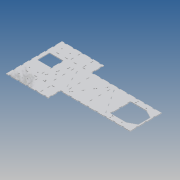
# Autodesk Inventor part: CaissonBase
Saved by Autodesk Inventor 2019 (Build 230136000, 136)
## iProperties
Created: 2019-08-26
Part Number: CaissonBase
Material: PVC-U
Document SubType Name: Modeling
Designer: jeremias.salamin
Density: 1.4 g/cm^3
Appearance: Lisse - Blanc
Description: CaissonBase
Mass: 70.9472 g
Surface Area: 655.131 cm^2
Volume: 50.6766 cm^3
Author: jeremias.salamin
Autodesk Inventor part; units mm, degrees
ref_plane "YZ Plane" through (0, 0, 0) normal (1, 0, 0) x (0, 1, 0)
ref_plane "XZ Plane" through (0, 0, 0) normal (0, 1, 0) x (-1, 0, 0)
ref_plane "XY Plane" through (0, 0, 0) normal (0, 0, 1) x (1, 0, 0)
sketch "Sketch1" plane through (0, 0, 0) normal (0, 0, 1) x (1, 0, 0)
  line L0 (0, 112) -> (0, -112) construction
  line L1 (-77.5006, 0) -> (370.4994, 0) construction
  line L2 (-13.5006, 0) -> (-13.5006, -80)
  line L3 (-13.5006, -80) -> (106.4994, -80)
  line L4 (106.4994, -80) -> (106.4994, -45)
  line L5 (106.4994, -45) -> (306.4994, -45)
  line L6 (306.4994, -45) -> (306.4994, 0)
  line L7 (-13.5006, 0) -> (-13.5006, 80)
  line L8 (-13.5006, 80) -> (106.4994, 80)
  line L9 (106.4994, 80) -> (106.4994, 45)
  line L10 (106.4994, 45) -> (306.4994, 45)
  line L11 (306.4994, 45) -> (306.4994, 0)
  point P0 (0, 0)
  dimension "d0" = 13.5006
  dimension "d1" = 80
  dimension "d2" = 120
  dimension "d3" = 200
  dimension "d4" = 45
  dimension "d5" = 320
  constraints: 20 end point, 4 symmetric about line, 2 perpendicular, 2 point on line, 1 parallel, 1 vertical
  measures "d0" distance between parallel lines of L7 L0
  measures "d1" distance of L2.start L2.end
  measures "d2" distance of L2.end L3.end
  measures "d3" distance of L4.end L5.end
  measures "d4" distance of L5.end L6.end
  measures "d5" distance between parallel lines of L2 L6
extrude "Extrusion1" add sketch "Sketch1" along normal mid plane 1.6
sketch "Esquisse2" plane through (0, 0, 0.8) normal (0, 0, 1) x (1, 0, 0)
  line L0 (-13.5006, 80) -> (-13.5006, -80) construction
  line L1 (-13.5006, -80) -> (106.4994, -80) construction
  line L2 (106.4994, -80) -> (106.4994, -45) construction
  line L3 (106.4994, -45) -> (306.4994, -45) construction
  line L4 (306.4994, -45) -> (306.4994, 45) construction
  line L5 (306.4994, 45) -> (106.4994, 45) construction
  line L6 (106.4994, 45) -> (106.4994, 80) construction
  line L7 (106.4994, 80) -> (-13.5006, 80) construction
  line L8 (0, 112) -> (0, -112) construction
  line L9 (-77.5006, 0) -> (370.4994, 0) construction
  arc A0 (278.9561, 15.2899) -> (278.9561, -15.2899) centre (255.4994, 0) ccw construction
  arc A1 (278.9561, -15.2899) -> (278.9561, 15.2899) centre (281.4994, 0) ccw construction
  line L10 (234.4994, 29.5) -> (279.4994, 29.5)
  line L11 (279.4994, -29.5) -> (234.4994, -29.5)
  line L12 (234.4994, -29.5) -> (234.4994, 29.5)
  line L13 (302.4994, -17.5) -> (302.4994, 17.5)
  line L14 (279.4994, 29.5) -> (302.4994, 17.5)
  line L15 (302.4994, -17.5) -> (279.4994, -29.5)
  point P0 (0, 0)
  dimension "d8" = 56
  dimension "d9" = 31
  dimension "d10" = 26
  dimension "d11" = 25
  dimension "d12" = 59
  dimension "d13" = 35
  dimension "d15" = 45
  dimension "d16" = 4
  dimension "d23" = 117.553
  dimension "d24" = 117.553
  dimension "d25" = 25.9422
  dimension "d62" = 27
  constraints: 12 end point, 4 point on circle, 2 centre point, 2 point on line, 1 horizontal, 1 parallel, 1 other
  measures "d8" diameter of A0
  measures "d9" diameter of A1
  measures "d10" distance of A1.centre A0.centre
  measures "d11" distance from line of L4 A1.centre
  measures "d12" distance of L11.end L10.start
  measures "d13" distance of L13.start L13.end
  measures "d15" distance of L10.start L10.end
  measures "d16" distance between parallel lines of L4 L13
  measures "d23" angle of L13 L14
  measures "d24" angle of L13 L15
  measures "d25" distance of L13.start L11.start
  measures "d62" distance from line of L4 L10.end
extrude "Extrusion2" cut sketch "Esquisse2" against normal through all
sketch "Esquisse3" plane through (0, 0, 0.8) normal (0, 0, 1) x (1, 0, 0)
  line L0 (234.4994, -29.5) -> (234.4994, 29.5) construction
  line L1 (234.4994, 29.5) -> (279.4994, 29.5) construction
  line L2 (279.4994, 29.5) -> (302.4994, 17.5) construction
  line L3 (302.4994, 17.5) -> (302.4994, -17.5) construction
  line L4 (302.4994, -17.5) -> (279.4994, -29.5) construction
  line L5 (279.4994, -29.5) -> (234.4994, -29.5) construction
  line L6 (-13.5006, 80) -> (-13.5006, -80) construction
  line L7 (-13.5006, -80) -> (106.4994, -80) construction
  line L8 (106.4994, -80) -> (106.4994, -45) construction
  line L9 (106.4994, -45) -> (306.4994, -45) construction
  line L10 (306.4994, -45) -> (306.4994, 45) construction
  line L11 (306.4994, 45) -> (106.4994, 45) construction
  line L12 (106.4994, 45) -> (106.4994, 80) construction
  line L13 (106.4994, 80) -> (-13.5006, 80) construction
  line L14 (0, 112) -> (0, -112) construction
  line L15 (-77.5006, 0) -> (370.4994, 0) construction
  point P0 (0, 0)
  point P1 (272.9994, 35)
  point P2 (272.9994, -35)
  dimension "d26" = 33.5
  dimension "d45" = 70
  constraints: 1 symmetric about line
  measures "d26" distance from line of point (272.999, 35) L10
  measures "d45" distance of point (272.999, -35) point (272.999, 35)
hole "Perçage3" at (272.9994, 35, 0.8) at (272.9994, -35, 0.8) direction (0, 0, -1) diameter 3 end through all
sketch "Esquisse4" plane through (0, 0, 0.8) normal (0, 0, 1) x (1, 0, 0)
  circle A0 centre (272.9994, 35) radius 1.5 construction
  circle A1 centre (272.9994, -35) radius 1.5 construction
  line L0 (234.4994, -29.5) -> (234.4994, 29.5) construction
  line L1 (234.4994, 29.5) -> (279.4994, 29.5) construction
  line L2 (279.4994, 29.5) -> (302.4994, 17.5) construction
  line L3 (302.4994, 17.5) -> (302.4994, -17.5) construction
  line L4 (302.4994, -17.5) -> (279.4994, -29.5) construction
  line L5 (279.4994, -29.5) -> (234.4994, -29.5) construction
  line L6 (-13.5006, 80) -> (-13.5006, -80) construction
  line L7 (-13.5006, -80) -> (106.4994, -80) construction
  line L8 (106.4994, -80) -> (106.4994, -45) construction
  line L9 (106.4994, -45) -> (306.4994, -45) construction
  line L10 (306.4994, -45) -> (306.4994, 45) construction
  line L11 (306.4994, 45) -> (106.4994, 45) construction
  line L12 (106.4994, 45) -> (106.4994, 80) construction
  line L13 (106.4994, 80) -> (-13.5006, 80) construction
  line L14 (0, 112) -> (0, -112) construction
  line L15 (-77.5006, 0) -> (370.4994, 0) construction
  line L16 (-3.5006, 34) -> (36.4994, 34)
  line L17 (36.4994, 34) -> (36.4994, -1.4)
  line L18 (36.4994, -1.4) -> (-3.5006, -1.4)
  line L19 (-3.5006, -1.4) -> (-3.5006, 34)
  point P0 (0, 0)
  dimension "d56" = 35.4
  dimension "d57" = 78.6
  dimension "d58" = 10
  dimension "d59" = 40
  constraints: 8 end point, 2 parallel, 1 horizontal, 1 perpendicular
  measures "d56" distance between parallel lines of L16 L18
  measures "d57" distance between parallel lines of L7 L18
  measures "d58" distance between parallel lines of L6 L19
  measures "d59" distance between parallel lines of L17 L19
extrude "Extrusion3" cut sketch "Esquisse4" against normal through all
sketch "Esquisse5" plane through (0, 0, 0.8) normal (0, 0, 1) x (1, 0, 0)
  line L0 (-3.5006, -1.4) -> (-3.5006, 34) construction
  line L1 (-3.5006, 34) -> (36.4994, 34) construction
  line L2 (36.4994, 34) -> (36.4994, -1.4) construction
  line L3 (36.4994, -1.4) -> (-3.5006, -1.4) construction
  circle A0 centre (272.9994, 35) radius 1.5 construction
  circle A1 centre (272.9994, -35) radius 1.5 construction
  line L4 (234.4994, -29.5) -> (234.4994, 29.5) construction
  line L5 (234.4994, 29.5) -> (279.4994, 29.5) construction
  line L6 (279.4994, 29.5) -> (302.4994, 17.5) construction
  line L7 (302.4994, 17.5) -> (302.4994, -17.5) construction
  line L8 (302.4994, -17.5) -> (279.4994, -29.5) construction
  line L9 (279.4994, -29.5) -> (234.4994, -29.5) construction
  line L10 (-13.5006, 80) -> (-13.5006, -80) construction
  line L11 (-13.5006, -80) -> (106.4994, -80) construction
  line L12 (106.4994, -80) -> (106.4994, -45) construction
  line L13 (106.4994, -45) -> (306.4994, -45) construction
  line L14 (306.4994, -45) -> (306.4994, 45) construction
  line L15 (306.4994, 45) -> (106.4994, 45) construction
  line L16 (106.4994, 45) -> (106.4994, 80) construction
  line L17 (106.4994, 80) -> (-13.5006, 80) construction
  line L18 (0, 112) -> (0, -112) construction
  line L19 (-77.5006, 0) -> (370.4994, 0) construction
  point P0 (0, 0)
  point P1 (4.4994, 61.4)
  point P2 (28.4994, 61.4)
  point P3 (4.4994, -61.4)
  point P4 (28.4994, -61.4)
  point P5 (4.4994, -31.4)
  point P6 (28.4994, -31.4)
  dimension "d63" = 18.6
  dimension "d64" = 18.6
  dimension "d65" = 24
  dimension "d66" = 18
  dimension "d67" = 30
  dimension "d68" = 30
  dimension "d69" = 24
  dimension "d70" = 18
  constraints: 2 symmetric about line
  measures "d63" distance from line of L17 point (4.499, 61.4)
  measures "d64" distance from line of L17 point (28.499, 61.4)
  measures "d65" distance of point (28.499, 61.4) point (4.499, 61.4)
  measures "d66" distance from line of point (4.499, 61.4) L10
  measures "d67" distance of point (4.499, -61.4) point (4.499, -31.4)
  measures "d68" distance of point (28.499, -61.4) point (28.499, -31.4)
  measures "d69" distance of point (4.499, -31.4) point (28.499, -31.4)
  measures "d70" distance from line of L10 point (4.499, -31.4)
hole "Perçage4" at (4.4994, 61.4, 0.8) at (28.4994, 61.4, 0.8) at (4.4994, -61.4, 0.8) at (28.4994, -61.4, 0.8) at (4.4994, -31.4, 0.8) at (28.4994, -31.4, 0.8) direction (0, 0, -1) diameter 3 end through all
sketch "Esquisse6" plane through (0, 0, 0.8) normal (0, 0, 1) x (1, 0, 0)
  circle A0 centre (4.4994, -31.4) radius 1.5 construction
  circle A1 centre (4.4994, -61.4) radius 1.5 construction
  circle A2 centre (4.4994, 61.4) radius 1.5 construction
  circle A3 centre (28.4994, 61.4) radius 1.5 construction
  circle A4 centre (28.4994, -61.4) radius 1.5 construction
  circle A5 centre (28.4994, -31.4) radius 1.5 construction
  line L0 (-3.5006, -1.4) -> (-3.5006, 34) construction
  line L1 (-3.5006, 34) -> (36.4994, 34) construction
  line L2 (36.4994, 34) -> (36.4994, -1.4) construction
  line L3 (36.4994, -1.4) -> (-3.5006, -1.4) construction
  circle A6 centre (272.9994, 35) radius 1.5 construction
  circle A7 centre (272.9994, -35) radius 1.5 construction
  line L4 (234.4994, -29.5) -> (234.4994, 29.5) construction
  line L5 (234.4994, 29.5) -> (279.4994, 29.5) construction
  line L6 (279.4994, 29.5) -> (302.4994, 17.5) construction
  line L7 (302.4994, 17.5) -> (302.4994, -17.5) construction
  line L8 (302.4994, -17.5) -> (279.4994, -29.5) construction
  line L9 (279.4994, -29.5) -> (234.4994, -29.5) construction
  line L10 (-13.5006, 80) -> (-13.5006, -80) construction
  line L11 (-13.5006, -80) -> (106.4994, -80) construction
  line L12 (106.4994, -80) -> (106.4994, -45) construction
  line L13 (106.4994, -45) -> (306.4994, -45) construction
  line L14 (306.4994, -45) -> (306.4994, 45) construction
  line L15 (306.4994, 45) -> (106.4994, 45) construction
  line L16 (106.4994, 45) -> (106.4994, 80) construction
  line L17 (106.4994, 80) -> (-13.5006, 80) construction
  line L18 (0, 112) -> (0, -112) construction
  line L19 (-77.5006, 0) -> (370.4994, 0) construction
  point P0 (0, 0)
  point P1 (244.4994, 40)
  point P2 (244.4994, -40)
  dimension "d78" = 5
  dimension "d79" = 62
  constraints: 1 symmetric about line
  measures "d78" distance from line of L15 point (244.499, 40)
  measures "d79" distance from line of L14 point (244.499, 40)
hole "Perçage5" at (244.4994, 40, 0.8) at (244.4994, -40, 0.8) direction (0, 0, -1) diameter 3 end through all
sketch "Esquisse7" plane through (0, 0, 0.8) normal (0, 0, 1) x (1, 0, 0)
  circle A0 centre (244.4994, 40) radius 1.5 construction
  circle A1 centre (244.4994, -40) radius 1.5 construction
  circle A2 centre (4.4994, -31.4) radius 1.5 construction
  circle A3 centre (4.4994, -61.4) radius 1.5 construction
  circle A4 centre (4.4994, 61.4) radius 1.5 construction
  circle A5 centre (28.4994, 61.4) radius 1.5 construction
  circle A6 centre (28.4994, -61.4) radius 1.5 construction
  circle A7 centre (28.4994, -31.4) radius 1.5 construction
  line L0 (-3.5006, -1.4) -> (-3.5006, 34) construction
  line L1 (-3.5006, 34) -> (36.4994, 34) construction
  line L2 (36.4994, 34) -> (36.4994, -1.4) construction
  line L3 (36.4994, -1.4) -> (-3.5006, -1.4) construction
  circle A8 centre (272.9994, 35) radius 1.5 construction
  circle A9 centre (272.9994, -35) radius 1.5 construction
  line L4 (234.4994, -29.5) -> (234.4994, 29.5) construction
  line L5 (234.4994, 29.5) -> (279.4994, 29.5) construction
  line L6 (279.4994, 29.5) -> (302.4994, 17.5) construction
  line L7 (302.4994, 17.5) -> (302.4994, -17.5) construction
  line L8 (302.4994, -17.5) -> (279.4994, -29.5) construction
  line L9 (279.4994, -29.5) -> (234.4994, -29.5) construction
  line L10 (-13.5006, 80) -> (-13.5006, -80) construction
  line L11 (-13.5006, -80) -> (106.4994, -80) construction
  line L12 (106.4994, -80) -> (106.4994, -45) construction
  line L13 (106.4994, -45) -> (306.4994, -45) construction
  line L14 (306.4994, -45) -> (306.4994, 45) construction
  line L15 (306.4994, 45) -> (106.4994, 45) construction
  line L16 (106.4994, 45) -> (106.4994, 80) construction
  line L17 (106.4994, 80) -> (-13.5006, 80) construction
  line L18 (-77.5006, 0) -> (370.4994, 0) construction
  line L19 (0, 112) -> (0, -112) construction
  point P0 (0, 0)
  point P1 (244.4994, 33.4)
  point P2 (244.4994, -33.4)
  dimension "d87" = 11.6
  dimension "d88" = 62
  constraints: 1 symmetric about line
  measures "d87" distance from line of L15 point (244.499, 33.4)
  measures "d88" distance from line of L14 point (244.499, 33.4)
hole "Perçage6" at (244.4994, 33.4, 0.8) at (244.4994, -33.4, 0.8) direction (0, 0, -1) diameter 4 end through all
sketch "Esquisse10" plane through (0, 0, -0.8) normal (0, 0, -1) x (-1, 0, 0)
  line L0 (-75.4994, -80) -> (-75.4994, -78.4)
  line L1 (-75.4994, -78.4) -> (-67.4994, -78.4)
  line L2 (-67.4994, -78.4) -> (-67.4994, -80)
  line L3 (-67.4994, -80) -> (-75.4994, -80)
  line L4 (-25.4994, -80) -> (-25.4994, -78.4)
  line L5 (-25.4994, -78.4) -> (-17.4994, -78.4)
  line L6 (-17.4994, -78.4) -> (-17.4994, -80)
  line L7 (-17.4994, -80) -> (-25.4994, -80)
  line L8 (7.5006, -78.4) -> (7.5006, -80)
  line L9 (7.5006, -80) -> (-0.4994, -80)
  line L10 (-0.4994, -80) -> (-0.4994, -78.4)
  line L11 (-0.4994, -78.4) -> (7.5006, -78.4)
  line L12 (-50.4994, -80) -> (-50.4994, -78.4)
  line L13 (-50.4994, -78.4) -> (-42.4994, -78.4)
  line L14 (-42.4994, -78.4) -> (-42.4994, -80)
  line L15 (-42.4994, -80) -> (-50.4994, -80)
  line L16 (-100.4994, -80) -> (-100.4994, -78.4)
  line L17 (-100.4994, -78.4) -> (-92.4994, -78.4)
  line L18 (-92.4994, -78.4) -> (-92.4994, -80)
  line L19 (-92.4994, -80) -> (-100.4994, -80)
  line L20 (-255.7994, -43.4) -> (-255.7994, -45)
  line L21 (-255.7994, -45) -> (-263.7994, -45)
  line L22 (-263.7994, -45) -> (-263.7994, -43.4)
  line L23 (-263.7994, -43.4) -> (-255.7994, -43.4)
  line L24 (-205.7994, -43.4) -> (-205.7994, -45)
  line L25 (-205.7994, -45) -> (-213.7994, -45)
  line L26 (-213.7994, -45) -> (-213.7994, -43.4)
  line L27 (-213.7994, -43.4) -> (-205.7994, -43.4)
  line L28 (-155.7994, -43.4) -> (-155.7994, -45)
  line L29 (-155.7994, -45) -> (-163.7994, -45)
  line L30 (-163.7994, -45) -> (-163.7994, -43.4)
  line L31 (-163.7994, -43.4) -> (-155.7994, -43.4)
  line L32 (-105.7994, -43.4) -> (-105.7994, -45)
  line L33 (-105.7994, -45) -> (-113.7994, -45)
  line L34 (-113.7994, -45) -> (-113.7994, -43.4)
  line L35 (-113.7994, -43.4) -> (-105.7994, -43.4)
  line L36 (-55.7994, -43.4) -> (-55.7994, -45)
  line L37 (-55.7994, -45) -> (-63.7994, -45)
  line L38 (-63.7994, -45) -> (-63.7994, -43.4)
  line L39 (-63.7994, -43.4) -> (-55.7994, -43.4)
  line L40 (-5.7994, -43.4) -> (-5.7994, -45)
  line L41 (-5.7994, -45) -> (-13.7994, -45)
  line L42 (-13.7994, -45) -> (-13.7994, -43.4)
  line L43 (-13.7994, -43.4) -> (-5.7994, -43.4)
  line L44 (-30.7994, -43.4) -> (-30.7994, -45)
  line L45 (-30.7994, -45) -> (-38.7994, -45)
  line L46 (-38.7994, -45) -> (-38.7994, -43.4)
  line L47 (-38.7994, -43.4) -> (-30.7994, -43.4)
  line L48 (-80.7994, -43.4) -> (-80.7994, -45)
  line L49 (-80.7994, -45) -> (-88.7994, -45)
  line L50 (-88.7994, -45) -> (-88.7994, -43.4)
  line L51 (-88.7994, -43.4) -> (-80.7994, -43.4)
  line L52 (-130.7994, -43.4) -> (-130.7994, -45)
  line L53 (-130.7994, -45) -> (-138.7994, -45)
  line L54 (-138.7994, -45) -> (-138.7994, -43.4)
  line L55 (-138.7994, -43.4) -> (-130.7994, -43.4)
  line L56 (-180.7994, -43.4) -> (-180.7994, -45)
  line L57 (-180.7994, -45) -> (-188.7994, -45)
  line L58 (-188.7994, -45) -> (-188.7994, -43.4)
  line L59 (-188.7994, -43.4) -> (-180.7994, -43.4)
  line L60 (-230.7994, -43.4) -> (-230.7994, -45)
  line L61 (-230.7994, -45) -> (-238.7994, -45)
  line L62 (-238.7994, -45) -> (-238.7994, -43.4)
  line L63 (-238.7994, -43.4) -> (-230.7994, -43.4)
  line L64 (-280.7994, -43.4) -> (-280.7994, -45)
  line L65 (-280.7994, -45) -> (-288.7994, -45)
  line L66 (-288.7994, -45) -> (-288.7994, -43.4)
  line L67 (-288.7994, -43.4) -> (-280.7994, -43.4)
  line L68 (13.5006, 30.5) -> (11.9006, 30.5)
  line L69 (11.9006, 30.5) -> (11.9006, 38.5)
  line L70 (11.9006, 38.5) -> (13.5006, 38.5)
  line L71 (13.5006, 38.5) -> (13.5006, 30.5)
  line L72 (13.5006, -15.5) -> (11.9006, -15.5)
  line L73 (11.9006, -15.5) -> (11.9006, -7.5)
  line L74 (11.9006, -7.5) -> (13.5006, -7.5)
  line L75 (13.5006, -7.5) -> (13.5006, -15.5)
  line L76 (13.5006, -61.5) -> (11.9006, -61.5)
  line L77 (11.9006, -61.5) -> (11.9006, -53.5)
  line L78 (11.9006, -53.5) -> (13.5006, -53.5)
  line L79 (13.5006, -53.5) -> (13.5006, -61.5)
  line L80 (13.5006, -38.5) -> (11.9006, -38.5)
  line L81 (11.9006, -38.5) -> (11.9006, -30.5)
  line L82 (11.9006, -30.5) -> (13.5006, -30.5)
  line L83 (13.5006, -30.5) -> (13.5006, -38.5)
  line L84 (13.5006, 7.5) -> (11.9006, 7.5)
  line L85 (11.9006, 7.5) -> (11.9006, 15.5)
  line L86 (11.9006, 15.5) -> (13.5006, 15.5)
  line L87 (13.5006, 15.5) -> (13.5006, 7.5)
  line L88 (13.5006, 53.5) -> (11.9006, 53.5)
  line L89 (11.9006, 53.5) -> (11.9006, 61.5)
  line L90 (11.9006, 61.5) -> (13.5006, 61.5)
  line L91 (13.5006, 61.5) -> (13.5006, 53.5)
  line L92 (-104.8994, -75.7) -> (-106.4994, -75.7)
  line L93 (-106.4994, -75.7) -> (-106.4994, -67.7)
  line L94 (-106.4994, -67.7) -> (-104.8994, -67.7)
  line L95 (-104.8994, -67.7) -> (-104.8994, -75.7)
  line L96 (-104.8994, -55.7) -> (-106.4994, -55.7)
  line L97 (-106.4994, -55.7) -> (-106.4994, -47.7)
  line L98 (-106.4994, -47.7) -> (-104.8994, -47.7)
  line L99 (-104.8994, -47.7) -> (-104.8994, -55.7)
  line L100 (-304.8994, -4) -> (-306.4994, -4)
  line L101 (-306.4994, -4) -> (-306.4994, 4)
  line L102 (-306.4994, 4) -> (-304.8994, 4)
  line L103 (-304.8994, 4) -> (-304.8994, -4)
  line L104 (-304.8994, -29) -> (-306.4994, -29)
  line L105 (-306.4994, -29) -> (-306.4994, -21)
  line L106 (-306.4994, -21) -> (-304.8994, -21)
  line L107 (-304.8994, -21) -> (-304.8994, -29)
  line L108 (-304.8994, 21) -> (-306.4994, 21)
  line L109 (-306.4994, 21) -> (-306.4994, 29)
  line L110 (-306.4994, 29) -> (-304.8994, 29)
  line L111 (-304.8994, 29) -> (-304.8994, 21)
  line L112 (-255.7994, 45) -> (-255.7994, 43.4)
  line L113 (-255.7994, 43.4) -> (-263.7994, 43.4)
  line L114 (-263.7994, 43.4) -> (-263.7994, 45)
  line L115 (-263.7994, 45) -> (-255.7994, 45)
  line L116 (-205.7994, 45) -> (-205.7994, 43.4)
  line L117 (-205.7994, 43.4) -> (-213.7994, 43.4)
  line L118 (-213.7994, 43.4) -> (-213.7994, 45)
  line L119 (-213.7994, 45) -> (-205.7994, 45)
  line L120 (-155.7994, 45) -> (-155.7994, 43.4)
  line L121 (-155.7994, 43.4) -> (-163.7994, 43.4)
  line L122 (-163.7994, 43.4) -> (-163.7994, 45)
  line L123 (-163.7994, 45) -> (-155.7994, 45)
  line L124 (-105.7994, 45) -> (-105.7994, 43.4)
  line L125 (-105.7994, 43.4) -> (-113.7994, 43.4)
  line L126 (-113.7994, 43.4) -> (-113.7994, 45)
  line L127 (-113.7994, 45) -> (-105.7994, 45)
  line L128 (-55.7994, 45) -> (-55.7994, 43.4)
  line L129 (-55.7994, 43.4) -> (-63.7994, 43.4)
  line L130 (-63.7994, 43.4) -> (-63.7994, 45)
  line L131 (-63.7994, 45) -> (-55.7994, 45)
  line L132 (-5.7994, 45) -> (-5.7994, 43.4)
  line L133 (-5.7994, 43.4) -> (-13.7994, 43.4)
  line L134 (-13.7994, 43.4) -> (-13.7994, 45)
  line L135 (-13.7994, 45) -> (-5.7994, 45)
  line L136 (-30.7994, 45) -> (-30.7994, 43.4)
  line L137 (-30.7994, 43.4) -> (-38.7994, 43.4)
  line L138 (-38.7994, 43.4) -> (-38.7994, 45)
  line L139 (-38.7994, 45) -> (-30.7994, 45)
  line L140 (-80.7994, 45) -> (-80.7994, 43.4)
  line L141 (-80.7994, 43.4) -> (-88.7994, 43.4)
  line L142 (-88.7994, 43.4) -> (-88.7994, 45)
  line L143 (-88.7994, 45) -> (-80.7994, 45)
  line L144 (-130.7994, 45) -> (-130.7994, 43.4)
  line L145 (-130.7994, 43.4) -> (-138.7994, 43.4)
  line L146 (-138.7994, 43.4) -> (-138.7994, 45)
  line L147 (-138.7994, 45) -> (-130.7994, 45)
  line L148 (-180.7994, 45) -> (-180.7994, 43.4)
  line L149 (-180.7994, 43.4) -> (-188.7994, 43.4)
  line L150 (-188.7994, 43.4) -> (-188.7994, 45)
  line L151 (-188.7994, 45) -> (-180.7994, 45)
  line L152 (-230.7994, 45) -> (-230.7994, 43.4)
  line L153 (-230.7994, 43.4) -> (-238.7994, 43.4)
  line L154 (-238.7994, 43.4) -> (-238.7994, 45)
  line L155 (-238.7994, 45) -> (-230.7994, 45)
  line L156 (-280.7994, 45) -> (-280.7994, 43.4)
  line L157 (-280.7994, 43.4) -> (-288.7994, 43.4)
  line L158 (-288.7994, 43.4) -> (-288.7994, 45)
  line L159 (-288.7994, 45) -> (-280.7994, 45)
  line L160 (-104.8994, 47.7) -> (-106.4994, 47.7)
  line L161 (-106.4994, 47.7) -> (-106.4994, 55.7)
  line L162 (-106.4994, 55.7) -> (-104.8994, 55.7)
  line L163 (-104.8994, 55.7) -> (-104.8994, 47.7)
  line L164 (-104.8994, 67.7) -> (-106.4994, 67.7)
  line L165 (-106.4994, 67.7) -> (-106.4994, 75.7)
  line L166 (-106.4994, 75.7) -> (-104.8994, 75.7)
  line L167 (-104.8994, 75.7) -> (-104.8994, 67.7)
  line L168 (-75.4994, 78.4) -> (-75.4994, 80)
  line L169 (-75.4994, 80) -> (-67.4994, 80)
  line L170 (-67.4994, 80) -> (-67.4994, 78.4)
  line L171 (-67.4994, 78.4) -> (-75.4994, 78.4)
  line L172 (-25.4994, 78.4) -> (-25.4994, 80)
  line L173 (-25.4994, 80) -> (-17.4994, 80)
  line L174 (-17.4994, 80) -> (-17.4994, 78.4)
  line L175 (-17.4994, 78.4) -> (-25.4994, 78.4)
  line L176 (7.5006, 80) -> (7.5006, 78.4)
  line L177 (7.5006, 78.4) -> (-0.4994, 78.4)
  line L178 (-0.4994, 78.4) -> (-0.4994, 80)
  line L179 (-0.4994, 80) -> (7.5006, 80)
  line L180 (-50.4994, 78.4) -> (-50.4994, 80)
  line L181 (-50.4994, 80) -> (-42.4994, 80)
  line L182 (-42.4994, 80) -> (-42.4994, 78.4)
  line L183 (-42.4994, 78.4) -> (-50.4994, 78.4)
  line L184 (-100.4994, 78.4) -> (-100.4994, 80)
  line L185 (-100.4994, 80) -> (-92.4994, 80)
  line L186 (-92.4994, 80) -> (-92.4994, 78.4)
  line L187 (-92.4994, 78.4) -> (-100.4994, 78.4)
  line L188 (-44.6994, 75.7) -> (-43.0994, 75.7)
  line L189 (-43.0994, 75.7) -> (-43.0994, 67.7)
  line L190 (-43.0994, 67.7) -> (-44.6994, 67.7)
  line L191 (-44.6994, 67.7) -> (-44.6994, 75.7)
  line L192 (-44.6994, 55.7) -> (-43.0994, 55.7)
  line L193 (-43.0994, 55.7) -> (-43.0994, 47.7)
  line L194 (-43.0994, 47.7) -> (-44.6994, 47.7)
  line L195 (-44.6994, 47.7) -> (-44.6994, 55.7)
  line L196 (-81.2994, 75.7) -> (-79.6994, 75.7)
  line L197 (-79.6994, 75.7) -> (-79.6994, 67.7)
  line L198 (-79.6994, 67.7) -> (-81.2994, 67.7)
  line L199 (-81.2994, 67.7) -> (-81.2994, 75.7)
  line L200 (-81.2994, 55.7) -> (-79.6994, 55.7)
  line L201 (-79.6994, 55.7) -> (-79.6994, 47.7)
  line L202 (-79.6994, 47.7) -> (-81.2994, 47.7)
  line L203 (-81.2994, 47.7) -> (-81.2994, 55.7)
  line L204 (-93.3693, 4.9446) -> (-91.9076, 4.2939)
  line L205 (-91.9076, 4.2939) -> (-95.1615, -3.0145)
  line L206 (-95.1615, -3.0145) -> (-96.6232, -2.3637)
  line L207 (-96.6232, -2.3637) -> (-93.3693, 4.9446)
  line L208 (-83.2009, 27.7833) -> (-81.7392, 27.1325)
  line L209 (-81.7392, 27.1325) -> (-84.9931, 19.8241)
  line L210 (-84.9931, 19.8241) -> (-86.4548, 20.4749)
  line L211 (-86.4548, 20.4749) -> (-83.2009, 27.7833)
  line L212 (-103.5377, -17.894) -> (-102.0761, -18.5448)
  line L213 (-102.0761, -18.5448) -> (-105.3299, -25.8531)
  line L214 (-105.3299, -25.8531) -> (-106.7916, -25.2024)
  line L215 (-106.7916, -25.2024) -> (-103.5377, -17.894)
  line L216 (-72.2994, 4) -> (-70.6994, 4)
  line L217 (-70.6994, 4) -> (-70.6994, -4)
  line L218 (-70.6994, -4) -> (-72.2994, -4)
  line L219 (-72.2994, -4) -> (-72.2994, 4)
  line L220 (-72.2994, 29) -> (-70.6994, 29)
  line L221 (-70.6994, 29) -> (-70.6994, 21)
  line L222 (-70.6994, 21) -> (-72.2994, 21)
  line L223 (-72.2994, 21) -> (-72.2994, 29)
  line L224 (-72.2994, -21) -> (-70.6994, -21)
  line L225 (-70.6994, -21) -> (-70.6994, -29)
  line L226 (-70.6994, -29) -> (-72.2994, -29)
  line L227 (-72.2994, -29) -> (-72.2994, -21)
  line L228 (-52.4477, -3.9304) -> (-53.9605, -4.4513)
  line L229 (-53.9605, -4.4513) -> (-56.5651, 3.1128)
  line L230 (-56.5651, 3.1128) -> (-55.0522, 3.6337)
  line L231 (-55.0522, 3.6337) -> (-52.4477, -3.9304)
  line L232 (-44.3085, -27.5684) -> (-45.8213, -28.0893)
  line L233 (-45.8213, -28.0893) -> (-48.4259, -20.5251)
  line L234 (-48.4259, -20.5251) -> (-46.913, -20.0042)
  line L235 (-46.913, -20.0042) -> (-44.3085, -27.5684)
  line L236 (-60.5869, 19.7076) -> (-62.0997, 19.1866)
  line L237 (-62.0997, 19.1866) -> (-64.7043, 26.7508)
  line L238 (-64.7043, 26.7508) -> (-63.1914, 27.2717)
  line L239 (-63.1914, 27.2717) -> (-60.5869, 19.7076)
  line L240 (-38.0994, 4) -> (-36.4994, 4)
  line L241 (-36.4994, 4) -> (-36.4994, -4)
  line L242 (-36.4994, -4) -> (-38.0994, -4)
  line L243 (-38.0994, -4) -> (-38.0994, 4)
  line L244 (-38.0994, 29) -> (-36.4994, 29)
  line L245 (-36.4994, 29) -> (-36.4994, 21)
  line L246 (-36.4994, 21) -> (-38.0994, 21)
  line L247 (-38.0994, 21) -> (-38.0994, 29)
  line L248 (-38.0994, -21) -> (-36.4994, -21)
  line L249 (-36.4994, -21) -> (-36.4994, -29)
  line L250 (-36.4994, -29) -> (-38.0994, -29)
  line L251 (-38.0994, -29) -> (-38.0994, -21)
  line L252 (-44.6994, -47.7) -> (-43.0994, -47.7)
  line L253 (-43.0994, -47.7) -> (-43.0994, -55.7)
  line L254 (-43.0994, -55.7) -> (-44.6994, -55.7)
  line L255 (-44.6994, -55.7) -> (-44.6994, -47.7)
  line L256 (-44.6994, -67.7) -> (-43.0994, -67.7)
  line L257 (-43.0994, -67.7) -> (-43.0994, -75.7)
  line L258 (-43.0994, -75.7) -> (-44.6994, -75.7)
  line L259 (-44.6994, -75.7) -> (-44.6994, -67.7)
  line L260 (-81.2994, -47.7) -> (-79.6994, -47.7)
  line L261 (-79.6994, -47.7) -> (-79.6994, -55.7)
  line L262 (-79.6994, -55.7) -> (-81.2994, -55.7)
  line L263 (-81.2994, -55.7) -> (-81.2994, -47.7)
  line L264 (-81.2994, -67.7) -> (-79.6994, -67.7)
  line L265 (-79.6994, -67.7) -> (-79.6994, -75.7)
  line L266 (-79.6994, -75.7) -> (-81.2994, -75.7)
  line L267 (-81.2994, -75.7) -> (-81.2994, -67.7)
  line L268 (-114.2994, -4) -> (-115.8994, -4)
  line L269 (-115.8994, -4) -> (-115.8994, 4)
  line L270 (-115.8994, 4) -> (-114.2994, 4)
  line L271 (-114.2994, 4) -> (-114.2994, -4)
  line L272 (-114.2994, -29) -> (-115.8994, -29)
  line L273 (-115.8994, -29) -> (-115.8994, -21)
  line L274 (-115.8994, -21) -> (-114.2994, -21)
  line L275 (-114.2994, -21) -> (-114.2994, -29)
  line L276 (-114.2994, 21) -> (-115.8994, 21)
  line L277 (-115.8994, 21) -> (-115.8994, 29)
  line L278 (-115.8994, 29) -> (-114.2994, 29)
  line L279 (-114.2994, 29) -> (-114.2994, 21)
  line L280 (-148.7608, 7.1952) -> (-150.1027, 6.3237)
  line L281 (-150.1027, 6.3237) -> (-154.4598, 13.0331)
  line L282 (-154.4598, 13.0331) -> (-153.1179, 13.9045)
  line L283 (-153.1179, 13.9045) -> (-148.7608, 7.1952)
  line L284 (-121.5288, -34.7384) -> (-122.8707, -35.6098)
  line L285 (-122.8707, -35.6098) -> (-127.2278, -28.9004)
  line L286 (-127.2278, -28.9004) -> (-125.8859, -28.029)
  line L287 (-125.8859, -28.029) -> (-121.5288, -34.7384)
  line L288 (-135.1448, -13.7716) -> (-136.4867, -14.643)
  line L289 (-136.4867, -14.643) -> (-140.8438, -7.9337)
  line L290 (-140.8438, -7.9337) -> (-139.5019, -7.0622)
  line L291 (-139.5019, -7.0622) -> (-135.1448, -13.7716)
  line L292 (-162.3768, 28.1619) -> (-163.7186, 27.2905)
  line L293 (-163.7186, 27.2905) -> (-168.0757, 33.9999)
  line L294 (-168.0757, 33.9999) -> (-166.7339, 34.8713)
  line L295 (-166.7339, 34.8713) -> (-162.3768, 28.1619)
  line L296 (-173.5994, -4) -> (-175.1994, -4)
  line L297 (-175.1994, -4) -> (-175.1994, 4)
  line L298 (-175.1994, 4) -> (-173.5994, 4)
  line L299 (-173.5994, 4) -> (-173.5994, -4)
  line L300 (-173.5994, -29) -> (-175.1994, -29)
  line L301 (-175.1994, -29) -> (-175.1994, -21)
  line L302 (-175.1994, -21) -> (-173.5994, -21)
  line L303 (-173.5994, -21) -> (-173.5994, -29)
  line L304 (-173.5994, 21) -> (-175.1994, 21)
  line L305 (-175.1994, 21) -> (-175.1994, 29)
  line L306 (-175.1994, 29) -> (-173.5994, 29)
  line L307 (-173.5994, 29) -> (-173.5994, 21)
  line L308 (-209.2969, -7.0622) -> (-207.955, -7.9337)
  line L309 (-207.955, -7.9337) -> (-212.3121, -14.643)
  line L310 (-212.3121, -14.643) -> (-213.654, -13.7716)
  line L311 (-213.654, -13.7716) -> (-209.2969, -7.0622)
  line L312 (-182.0649, 34.8713) -> (-180.7231, 33.9999)
  line L313 (-180.7231, 33.9999) -> (-185.0802, 27.2905)
  line L314 (-185.0802, 27.2905) -> (-186.422, 28.1619)
  line L315 (-186.422, 28.1619) -> (-182.0649, 34.8713)
  line L316 (-195.6809, 13.9045) -> (-194.339, 13.0331)
  line L317 (-194.339, 13.0331) -> (-198.6961, 6.3237)
  line L318 (-198.6961, 6.3237) -> (-200.038, 7.1952)
  line L319 (-200.038, 7.1952) -> (-195.6809, 13.9045)
  line L320 (-222.9129, -28.029) -> (-221.571, -28.9004)
  line L321 (-221.571, -28.9004) -> (-225.9281, -35.6098)
  line L322 (-225.9281, -35.6098) -> (-227.27, -34.7384)
  line L323 (-227.27, -34.7384) -> (-222.9129, -28.029)
  line L324 (-234.4994, 4) -> (-232.8994, 4)
  line L325 (-232.8994, 4) -> (-232.8994, -4)
  line L326 (-232.8994, -4) -> (-234.4994, -4)
  line L327 (-234.4994, -4) -> (-234.4994, 4)
  line L328 (-234.4994, 29) -> (-232.8994, 29)
  line L329 (-232.8994, 29) -> (-232.8994, 21)
  line L330 (-232.8994, 21) -> (-234.4994, 21)
  line L331 (-234.4994, 21) -> (-234.4994, 29)
  line L332 (-234.4994, -21) -> (-232.8994, -21)
  line L333 (-232.8994, -21) -> (-232.8994, -29)
  line L334 (-232.8994, -29) -> (-234.4994, -29)
  line L335 (-234.4994, -29) -> (-234.4994, -21)
  point P0 (0, 0)
  constraints: 672 end point, 140 horizontal, 140 vertical, 392 other
extrude "Extrusion5" cut sketch "Esquisse10" against normal blind 1.6
sketch "Esquisse11" plane through (0, 0, 0.8) normal (0, 0, 1) x (1, 0, 0)
  circle A0 centre (59.5084, -10.25) radius 1.7 projected
  circle A1 centre (59.5084, -40.25) radius 1.7 projected
  point P0 (0, 0)
extrude "Extrusion6" cut sketch "Esquisse11" against normal through all
equation "\"d21\" = d8"
